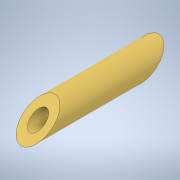
# Autodesk Inventor part: Maccaroni
Saved by Autodesk Inventor 2021 (Build 250183000, 183)
## iProperties
Created: 2022-03-16
Part Number: Maccaroni
Material: Generic
Document SubType Name: Modeling
Designer: Lukas
Density: 1 g/cm^3
Appearance: Default
Author: Lukas
Autodesk Inventor part; units mm, degrees
ref_plane "YZ Plane" through (0, 0, 0) normal (1, 0, 0) x (0, 1, 0)
ref_plane "XZ Plane" through (0, 0, 0) normal (0, 1, 0) x (-1, 0, 0)
ref_plane "XY Plane" through (0, 0, 0) normal (0, 0, 1) x (1, 0, 0)
sketch "Sketch1" plane through (0, 0, 0) normal (0, 0, 1) x (1, 0, 0)
  circle A0 centre (0, 0) radius 2
  circle A1 centre (0, 0) radius 4.1
  dimension "d0" = 8.2
  dimension "d1" = 4
  constraints: 2 centre point, 2 coincident
  measures "d0" diameter of A1
  measures "d1" diameter of A0
extrude "Extrusion1" add sketch "Sketch1" along normal blind 40
sketch "Sketch2" plane through (0, 0, 0) normal (1, 0, 0) x (0, 1, 0)
  line L0 (4.1, 0) -> (4.1, 40) projected
  line L1 (-4.1, 0) -> (-4.1, 40) projected
  line L2 (4.1, 40) -> (-4.1, 40) projected
  line L3 (-4.1, 0) -> (4.1, 0) projected
  line L4 (-4.1, 40) -> (4.1, 30.2276)
  line L5 (4.1, 0) -> (-4.1, 9.7724)
  point P0 (0, 0)
  dimension "d4" = 40
  constraints: 4 end point, 2 point on line, 1 parallel
  measures "d4" angle of L1 L4
extrude "Extrusion2" cut sketch "Sketch2" along normal through all both and the other way through all contours L3 L1 L5 | L4 L2 L0
body "Solid1"
